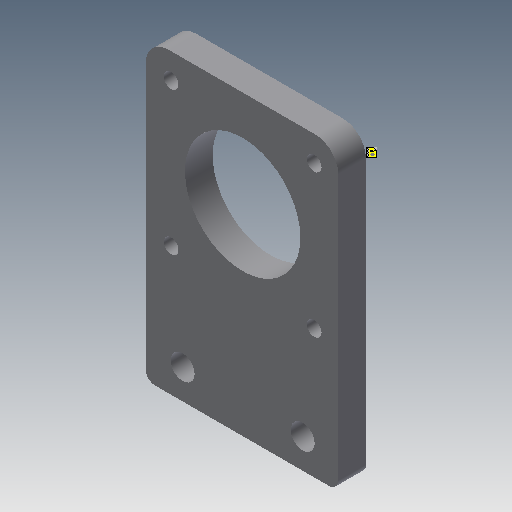
# Autodesk Inventor part: Z Motor Mount LC
Saved by Autodesk Inventor 2017 (Build 210142000, 142)
## iProperties
Created: 2016-06-20
Part Number: Z Motor Mount LC
Material: Generic
Document SubType Name: Modeling
Designer: joshmamo
Density: 1 g/cm^3
Appearance: Default
Author: joshmamo
Autodesk Inventor part; units mm, degrees
ref_plane "YZ Plane" through (0, 0, 0) normal (1, 0, 0) x (0, 1, 0)
ref_plane "XZ Plane" through (0, 0, 0) normal (0, 1, 0) x (-1, 0, 0)
ref_plane "XY Plane" through (0, 0, 0) normal (0, 0, 1) x (1, 0, 0)
sketch "Sketch1" plane through (0, 0, 0) normal (0, 0, 1) x (1, 0, 0)
  line L0 (2, -8.4394) -> (39.7013, -8.4394)
  line L1 (41.7013, 2) -> (41.7013, 48)
  line L2 (36.7013, 53) -> (5, 53)
  line L3 (0, 48) -> (0, 2)
  line L4 (5, 53) -> (36.7013, 53)
  line L5 (41.7013, 48) -> (41.7013, 11.2987)
  line L6 (0, 11) -> (0, 48)
  circle A0 centre (21, 32) radius 12.5
  circle A1 centre (5.5, 47.5) radius 1.6
  circle A2 centre (36.5, 47.5) radius 1.6
  circle A3 centre (36.5, 16.5) radius 1.6
  circle A4 centre (5.5, 16.5) radius 1.6
  line L7 (0, 2) -> (0, 5.5)
  circle A5 centre (34, -0.0146) radius 2.6
  circle A6 centre (8, -0.0146) radius 2.6
  arc A7 (5, 53) -> (0, 48) centre (5, 48) ccw
  arc A8 (41.7013, 48) -> (36.7013, 53) centre (36.7013, 48) ccw
  arc A9 (0, -6.4394) -> (2, -8.4394) centre (2, -6.4394) ccw
  arc A10 (39.7013, -8.4394) -> (41.7013, -6.4353) centre (39.7013, -6.4394) ccw
  line L8 (8, 53) -> (71, 53) construction
  line L9 (8, -15.5146) -> (8, 4.4854)
  line L10 (8, 10) -> (19.9253, 10)
  line L11 (19.9253, 10) -> (19.9253, 0)
  line L12 (41.7013, -6.4394) -> (41.7013, 2)
  line L13 (0, -6.4394) -> (0, 2)
  line L14 (19.9253, 0) -> (19.9253, -8.5)
  point P0 (0, 0)
  point P1 (41.7013, 0)
  dimension "d8" = 3.2
  dimension "d9" = 3.2
  dimension "d10" = 5.5
  dimension "d13" = 5.2
  dimension "d14" = 5.2
  dimension "d16" = 2
  dimension "d22" = 20
  dimension "d23" = 10
  dimension "d24" = 8.5
  constraints: 30 end point, 11 centre point, 9 point on circle, 6 tangent, 4 coincident, 4 parallel, 4 perpendicular, 4 point on line, 3 horizontal, 2 equal radius, 1 vertical
  measures "d8" diameter of A3
  measures "d9" diameter of A4
  measures "d10" distance of point (0, 0) L7.end
  measures "d13" diameter of A5
  measures "d14" diameter of A6
  measures "d16" radius of A9
  measures "d22" distance of L9.start L9.end
  measures "d23" distance of L10.end L11.end
  measures "d24" distance of L11.end L14.end
sketch "Sketch2" plane through (0, 0, 0) normal (0, 0, 1) x (1, 0, 0)
  circle A0 centre (21, 32) radius 12.5 projected
  line L0 (36.7013, 53) -> (5, 53) projected
  arc A1 (41.7013, 48) -> (36.7013, 53) centre (36.7013, 48) ccw projected
  line L1 (41.7013, -6.4353) -> (41.7013, 48) projected
  arc A2 (39.7013, -8.4394) -> (41.7013, -6.4353) centre (39.7013, -6.4394) ccw projected
  line L2 (2, -8.4394) -> (39.7013, -8.4394) projected
  arc A3 (0, -6.4394) -> (2, -8.4394) centre (2, -6.4394) ccw projected
  line L3 (0, 48) -> (0, -8.0248) projected
  arc A4 (5, 53) -> (0, 48) centre (5, 48) ccw projected
  circle A5 centre (5.5, 47.5) radius 1.6 projected
  circle A6 centre (36.5, 47.5) radius 1.6 projected
  circle A7 centre (36.5, 16.5) radius 1.6 projected
  circle A8 centre (5.5, 16.5) radius 1.6 projected
  circle A9 centre (8, -0.0146) radius 2.6 projected
  circle A10 centre (34, -0.0146) radius 2.6 projected
  line L4 (27.3496, 53) -> (27.3496, 13)
  line L5 (27.3496, 53) -> (67.3496, 53) construction
  line L6 (27.3496, 13) -> (27.3496, -7)
  line L7 (27.3496, -7) -> (27.3496, 3)
  line L8 (27.3496, 3) -> (19.3517, 3)
  point P0 (0, 0)
  dimension "d17" = 40
  dimension "d18" = 90
  dimension "d19" = 20
  constraints: 10 end point, 2 horizontal, 2 point on line, 1 midpoint, 1 perpendicular, 1 vertical, 1 other
  measures "d17" distance of L4.start L4.end
  measures "d18" angle of L4 L5
  measures "d19" distance of L4.end L6.end
sketch "Sketch3" plane through (0, 0, 0) normal (0, 0, 1) x (1, 0, 0)
  line L0 (36.7013, 53) -> (5, 53) projected
  arc A0 (41.7013, 48) -> (36.7013, 53) centre (36.7013, 48) ccw projected
  line L1 (41.7013, 2) -> (41.7013, 48) projected
  line L2 (41.7013, -6.4353) -> (41.7013, 2) projected
  arc A1 (39.7013, -8.4394) -> (41.7013, -6.4353) centre (39.7013, -6.4394) ccw projected
  line L3 (2, -8.4394) -> (39.7013, -8.4394) projected
  arc A2 (0, -6.4394) -> (2, -8.4394) centre (2, -6.4394) ccw projected
  line L4 (0, -8.0248) -> (0, 2) projected
  line L5 (0, 48) -> (0, 2) projected
  arc A3 (5, 53) -> (0, 48) centre (5, 48) ccw projected
  circle A4 centre (5.5, 47.5) radius 1.6 projected
  circle A5 centre (36.5, 47.5) radius 1.6 projected
  circle A6 centre (21, 32) radius 12.5 projected
  circle A7 centre (5.5, 16.5) radius 1.6 projected
  circle A8 centre (36.5, 16.5) radius 1.6 projected
  circle A9 centre (34, -0.0146) radius 2.6 projected
  circle A10 centre (8, -0.0146) radius 2.6 projected
  point P0 (0, 0)
  constraints: 1 other
sketch "Sketch4" plane through (0, 0, 0) normal (0, 0, 1) x (1, 0, 0)
  line L0 (36.7013, 58) -> (5, 58)
  arc A0 (41.7013, 53) -> (36.7013, 58) centre (36.7013, 53) ccw
  line L1 (41.7013, 2) -> (41.7013, 53)
  line L2 (0, -4.4394) -> (0, 2)
  line L3 (0, 2) -> (0, 5.5)
  line L4 (0, 53) -> (0, 2)
  arc A1 (5, 58) -> (0, 53) centre (5, 53) ccw
  circle A2 centre (5.5, 52.5) radius 1.6
  circle A3 centre (36.5, 52.5) radius 1.6
  circle A4 centre (21, 37) radius 12.5
  circle A5 centre (5.5, 21.5) radius 1.6
  circle A6 centre (36.5, 21.5) radius 1.6
  circle A7 centre (8, -0.0146) radius 2.6
  circle A8 centre (34, -0.0146) radius 2.6
  line L5 (41.7013, -4.4394) -> (41.7013, 2)
  line L6 (2, -6.4394) -> (39.7013, -6.4394)
  arc A9 (0, -4.4394) -> (2, -6.4394) centre (2, -4.4394) ccw
  arc A10 (39.7013, -6.4394) -> (41.7013, -4.4394) centre (39.7013, -4.4394) ccw
  line L7 (21, 37) -> (26, 37) construction
  point P0 (0, 0)
  point P1 (0, -6.4394)
  point P2 (41.7013, -6.4394)
  dimension "d27" = 2
  constraints: 16 end point, 11 centre point, 8 point on circle, 4 point on line, 4 tangent, 1 equal radius, 1 horizontal
  measures "d27" radius of A9
extrude "Extrusion1" add sketch "Sketch4" along normal blind 6
body "Solid1"
